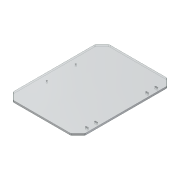
# Autodesk Inventor part: Clear Right Side Door
Saved by Autodesk Inventor 2015 (Build 190159000, 159)
## iProperties
Created: 2018-04-14
Part Number: Clear Right Side Door
Material: Glass
Document SubType Name: Modeling
Designer: Ghassan Yusuf
Density: 2.18 g/cm^3
Appearance: Clear
Author: Ghassan Yusuf
Autodesk Inventor part; units mm, degrees
ref_plane "YZ Plane" through (0, 0, 0) normal (1, 0, 0) x (0, 1, 0)
ref_plane "XZ Plane" through (0, 0, 0) normal (0, 1, 0) x (-1, 0, 0)
ref_plane "XY Plane" through (0, 0, 0) normal (0, 0, 1) x (1, 0, 0)
sketch "Hinges Screw Holes" plane through (0, 0, 0) normal (0, 0, 1) x (1, 0, 0)
  arc A0 (172, -72.429) -> (172, -68.929) centre (172, -70.679) ccw
  arc A1 (172, -97.929) -> (172, -94.429) centre (172, -96.179) ccw
  arc A2 (167, 97.929) -> (167, 94.429) centre (167, 96.179) ccw
  arc A3 (167, 72.429) -> (167, 68.929) centre (167, 70.679) ccw
  arc A4 (167, -68.929) -> (167, -72.429) centre (167, -70.679) ccw
  arc A5 (167, -94.429) -> (167, -97.929) centre (167, -96.179) ccw
  line L0 (167, 97.929) -> (172, 97.929)
  line L1 (167, 94.429) -> (172, 94.429)
  line L2 (167, 72.429) -> (172, 72.429)
  line L3 (167, 68.929) -> (172, 68.929)
  line L4 (167, -68.929) -> (172, -68.929)
  line L5 (167, -72.429) -> (172, -72.429)
  line L6 (167, -94.429) -> (172, -94.429)
  line L7 (167, -97.929) -> (172, -97.929)
  arc A6 (172, 94.429) -> (172, 97.929) centre (172, 96.179) ccw
  arc A7 (172, 68.929) -> (172, 72.429) centre (172, 70.679) ccw
  point P0 (169.5, 0)
  dimension "d28" = 3.5
  dimension "d29" = 3.5
  dimension "d30" = 25.5
  dimension "d31" = 3.5
  dimension "d32" = 3.5
  dimension "d33" = 25.5
  dimension "d34" = 141.358
  dimension "d35" = 3.5
  dimension "d36" = 3.5
  dimension "d37" = 25.5
  dimension "d38" = 3.5
  dimension "d39" = 3.5
  dimension "d40" = 25.5
  dimension "d41" = 141.358
  dimension "d42" = 5
  measures "d28" diameter of A6
  measures "d29" diameter of A7
  measures "d30" distance of A7.centre A6.centre
  measures "d31" diameter of A0
  measures "d32" diameter of A1
  measures "d33" distance of A1.centre A0.centre
  measures "d34" distance of A0.centre A7.centre
  measures "d35" diameter of A2
  measures "d36" diameter of A3
  measures "d37" distance of A3.centre A2.centre
  measures "d38" diameter of A4
  measures "d39" diameter of A5
  measures "d40" distance of A5.centre A4.centre
  measures "d41" distance of A4.centre A3.centre
  measures "d42" distance of A6.centre A2.centre
sketch "Handle-Hole" plane through (0, 0, 0) normal (0, 0, 1) x (1, 0, 0)
  line L0 (-99.5, 50) -> (-69.5, 50)
  line L1 (-69.5, 50) -> (-69.5, -50)
  line L2 (-69.5, -50) -> (-99.5, -50)
  line L3 (-99.5, -50) -> (-99.5, 50)
  circle A0 centre (-87.5, 62) radius 1.75
  circle A1 centre (-57.5, 27.5) radius 1.75
  circle A2 centre (-57.5, -27.5) radius 1.75
  circle A3 centre (-87.5, -62) radius 1.75
  point P0 (-82.2826, 0)
  point P1 (-99.5, 0)
  point P2 (-99.5, 0)
  dimension "d11" = 30
  dimension "d12" = 100
  dimension "d13" = 3.5
  dimension "d14" = 3.5
  dimension "d15" = 3.5
  dimension "d16" = 3.5
  dimension "d17" = 55
  dimension "d19" = 12
  dimension "d20" = 12
  dimension "d22" = 12
  measures "d11" distance of L1.end L2.end
  measures "d12" distance of L0.end L1.end
  measures "d13" diameter of A0
  measures "d14" diameter of A1
  measures "d15" diameter of A2
  measures "d16" diameter of A3
  measures "d17" distance of A2.centre A1.centre
  measures "d19" distance from line of L2 A3.centre
  measures "d20" distance from line of L0 A0.centre
  measures "d22" distance from line of L1 A1.centre
sketch "Sketch1" plane through (0, 0, 0) normal (0, 0, 1) x (1, 0, 0)
  line L0 (-100, 133.5) -> (100, 133.5)
  line L1 (100, 133.5) -> (100, -133.5)
  line L2 (100, -133.5) -> (-100, -133.5)
  line L3 (-100, -133.5) -> (-100, 133.5)
  line L4 (99.5, 133) -> (-99.5, 133)
  line L5 (-99.5, 133) -> (-99.5, -133)
  line L6 (-99.5, -133) -> (99.5, -133)
  line L7 (99.5, -133) -> (99.5, 133)
  point P0 (0, 0)
  point P1 (0, 133.5)
  point P2 (-99.5, 0)
  dimension "d0" = 200
  dimension "d1" = 267
  dimension "d4" = 0.5
  constraints: 16 end point, 4 parallel, 2 midpoint, 2 perpendicular, 1 horizontal, 1 horizontal alignment, 1 vertical alignment, 3 other
  measures "d0" distance of L1.end L2.end
  measures "d1" distance of L0.end L1.end
  measures "d4" distance between parallel lines of L0 L4
extrude "Extrusion1" add sketch "Sketch1" along normal blind 5 contours L7 L6 L5 L4
chamfer "Chamfer1" distance 20 angle 45 4 edges at (-99.5, -133, 2.5) (-99.5, 133, 2.5) (99.5, -133, 2.5) (99.5, 133, 2.5)
fillet "Fillet1" radius 5 8 edges at (-79.5, -133, 2.5) (79.5, -133, 2.5) (99.5, -113, 2.5) (99.5, 113, 2.5) (79.5, 133, 2.5) (-79.5, 133, 2.5) (-99.5, 113, 2.5) (-99.5, -113, 2.5)
sketch "Sketch2" plane through (0, 0, 5) normal (0, 0, 1) x (1, 0, 0)
  line L0 (99.5, -110.9289) -> (99.5, 110.9289) projected
  circle A0 centre (-79.5, 40) radius 1.75
  circle A1 centre (-79.5, -40) radius 1.75
  line L1 (-99.5, 110.9289) -> (-99.5, -110.9289) projected
  arc A2 (90, -72.429) -> (90, -68.929) centre (90, -70.679) ccw
  arc A3 (90, -97.929) -> (90, -94.429) centre (90, -96.179) ccw
  arc A4 (85, 97.929) -> (85, 94.429) centre (85, 96.179) ccw
  arc A5 (85, 72.429) -> (85, 68.929) centre (85, 70.679) ccw
  arc A6 (85, -68.929) -> (85, -72.429) centre (85, -70.679) ccw
  arc A7 (85, -94.429) -> (85, -97.929) centre (85, -96.179) ccw
  line L2 (85, 97.929) -> (90, 97.929)
  line L3 (85, 94.429) -> (90, 94.429)
  line L4 (85, 72.429) -> (90, 72.429)
  line L5 (85, 68.929) -> (90, 68.929)
  line L6 (85, -68.929) -> (90, -68.929)
  line L7 (85, -72.429) -> (90, -72.429)
  line L8 (85, -94.429) -> (90, -94.429)
  line L9 (85, -97.929) -> (90, -97.929)
  arc A8 (90, 94.429) -> (90, 97.929) centre (90, 96.179) ccw
  arc A9 (90, 68.929) -> (90, 72.429) centre (90, 70.679) ccw
  point P0 (0, 0)
  point P1 (0, 0)
  dimension "d43" = 141.358
  dimension "d44" = 70.679
  dimension "d45" = 9.5
  dimension "d46" = 9.5
  dimension "d47" = 3.5
  dimension "d48" = 80
  dimension "d49" = 20
  dimension "d50" = 40
  constraints: 2 centre point, 1 equal radius, 1 vertical alignment
  measures "d47" diameter of A0
  measures "d48" distance of A1.centre A0.centre
  measures "d49" distance from line of L1 A0.centre
  measures "d50" vertical distance of point (0, 0) A0.centre
extrude "Extrusion2" cut sketch "Sketch2" against normal blind 10
equation "\"d44\" = 0.5 * d43"
equation "\"d50\" = 0.5 * d48"
equation "\"d19\" = d20"
equation "\"d20\" = d21"
equation "\"d22\" = d21"
equation "\"d46\" = d45"
equation "\"d21\" = 12"
body "Solid1"
